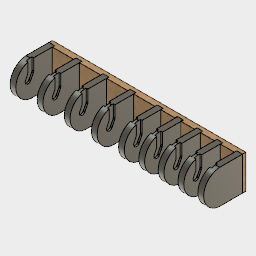
NEW AND IMPROVED Spool Holder x8 v3 (Autodesk Fusion 360 design; units mm, degrees)
Autodesk Fusion 360 part; units mm, degrees
note: some values were not read from the file. Chosen so that the rebuilt part matches the saved one: which face or edge a step refers to. Set by a fixed rule: which sketch regions a step uses.
sketch "Sketch1" plane through (0, 0, 0) normal (0, 1, 0) x (1, 0, 0)
  line L0 (-70, -30) -> (318, -30)
  line L1 (318, -30) -> (318, 40)
  line L2 (318, 40) -> (-70, 40)
  line L3 (-70, 40) -> (-70, -30)
  dimension "d1" = 70
  dimension "d2" = 388
  measures "d1" distance of L0.start L2.end
  measures "d2" distance of L0.start L0.end
extrude "Extrude1" add sketch "Sketch1" along normal blind 9 makes body 1
sketch "Sketch2" plane through (0, 0, 0) normal (0, -1, 0) x (1, 0, 0)
  line L0 (-70, 30) -> (-70, -40)
  line L1 (-70, 30) -> (-64, 30)
  line L2 (-64, 30) -> (-64, -40)
  line L3 (-64, -40) -> (-70, -40)
  line L4 (-70, -40) -> (-70, 30)
  line L5 (-20, 30) -> (-8, 30)
  line L6 (-8, 30) -> (-8, -40)
  line L7 (-8, -40) -> (-20, -40)
  line L8 (-20, -40) -> (-20, 30)
  line L9 (-70, 30) -> (318, 30)
  line L10 (318, -40) -> (-70, -40)
  line L11 (36, 30) -> (48, 30)
  line L12 (48, 30) -> (48, -40)
  line L13 (48, -40) -> (36, -40)
  line L14 (36, -40) -> (36, 30)
  line L15 (92, 30) -> (104, 30)
  line L16 (104, 30) -> (104, -40)
  line L17 (104, -40) -> (92, -40)
  line L18 (92, -40) -> (92, 30)
  line L19 (148, 30) -> (160, 30)
  line L20 (160, 30) -> (160, -40)
  line L21 (160, -40) -> (148, -40)
  line L22 (148, -40) -> (148, 30)
  line L23 (189, 30) -> (201, 30)
  line L24 (201, 30) -> (201, -40)
  line L25 (201, -40) -> (189, -40)
  line L26 (189, -40) -> (189, 30)
  line L27 (230, 30) -> (242, 30)
  line L28 (242, 30) -> (242, -40)
  line L29 (242, -40) -> (230, -40)
  line L30 (230, -40) -> (230, 30)
  line L31 (271, 30) -> (283, 30)
  line L32 (283, 30) -> (283, -40)
  line L33 (283, -40) -> (271, -40)
  line L34 (271, -40) -> (271, 30)
  line L35 (312, 30) -> (318, 30)
  line L36 (318, 30) -> (318, -40)
  line L37 (318, -40) -> (312, -40)
  line L38 (312, -40) -> (312, 30)
  dimension "d15" = 6
  dimension "d22" = 12
  dimension "d23" = 12
  dimension "d24" = 12
  dimension "d25" = 12
  dimension "d26" = 12
  dimension "d27" = 44
  dimension "d28" = 44
  dimension "d29" = 44
  dimension "d30" = 44
  dimension "d31" = 29
  dimension "d32" = 29
  dimension "d33" = 29
  dimension "d34" = 12
  dimension "d35" = 12
  dimension "d36" = 6
  dimension "d37" = 29
  measures "d15" distance of L0.start L1.end
  measures "d22" distance of L5.start L5.end
  measures "d23" distance of L11.start L11.end
  measures "d24" distance of L15.start L15.end
  measures "d25" distance of L19.start L19.end
  measures "d26" distance of L23.start L23.end
  measures "d27" distance of L2 L8
  measures "d28" distance of L6 L14
  measures "d29" distance of L12 L18
  measures "d30" distance of L16 L22
  measures "d31" distance of L20 L26
  measures "d32" distance of L24 L30
  measures "d33" distance of L28 L34
  measures "d34" distance of L28 L30
  measures "d35" distance of L32 L34
  measures "d36" distance of L36 L38
  measures "d37" distance of L32 L38
extrude "Extrude2" cut sketch "Sketch2" against normal blind 5 contours L0 L1 L2 L3 L4 L9 L10 | L5 L6 L7 L8 L9 L10 | L9 L10 L11 L12 L13 L14 | L9 L10 L15 L16 L17 L18 | L9 L10 L19 L20 L21 L22 | L9 L10 L23 L24 L25 L26 | L9 L10 L27 L28 L29 L30 | L9 L10 L31 L32 L33 L34 | L9 L10 L35 L36 L37 L38 bodies 1
extrude "Extrude3" add 1 faces at (-68, 5, -16.6667) along direction (0, -1, 0) blind 100 separate body on bodies 1 makes body 2
sketch "Sketch3" plane through (0, 5, 0) normal (0, -1, 0) x (1, 0, 0)
  line L0 (-8, 30) -> (-20, 30)
  line L1 (-20, 30) -> (-20, -40)
  line L2 (-20, -40) -> (-8, -40)
  line L3 (-8, -40) -> (-8, 30)
  line L4 (-14, 30) -> (-14, -40)
sketch "Sketch4" plane through (-70, 0, 0) normal (-1, 0, 0) x (0, -1, 0)
  line L0 (-5, 30) -> (-5, -40)
  line L1 (-5, -40) -> (95, -40)
  line L2 (95, -40) -> (95, 30)
  line L3 (95, 30) -> (-5, 30)
  line L4 (0, 30) -> (0, -40)
  line L5 (0, -5) -> (44.9994, -5.2262)
  circle A0 centre (44.9994, -5.2262) radius 40
  circle A1 centre (40, -5.1131) radius 35.1778
  point P0 (0, 30)
  point P1 (0, -40)
  dimension "d46" = 45
  dimension "d47" = 80
  dimension "d48" = 40
  measures "d46" distance of L5.start L5.end
  measures "d47" diameter of A0
  measures "d48" distance of L4 A1.centre
extrude "Extrude5" cut sketch "Sketch4" against normal blind 6 contours L1 L3 A0 A1 | L1 L2 L3 A0 picked at (81.0139, 1.7538) bodies 2
sketch "Sketch6" plane through (-70, 0, 0) normal (-1, 0, 0) x (0, -1, 0)
  arc A0 (44.5145, -40) -> (42.133, 30) centre (40, -5.1131) ccw
  line L0 (42.133, 30) -> (-5, 30)
  line L1 (-5, 30) -> (-5, -40)
  line L2 (-5, -40) -> (44.5145, -40)
  line L3 (-5, -5) -> (40, -5)
  circle A1 centre (40, -5) radius 2.5
  dimension "d53" = 45
  dimension "d54" = 5
  measures "d53" distance of L3.start L3.end
  measures "d54" diameter of A1
sketch "Sketch7" plane through (-64, 0, 0) normal (1, 0, 0) x (0, 1, 0)
  arc A0 (-42.133, 30) -> (-44.5145, -40) centre (-40, -5.1131) ccw
  line L0 (-44.5145, -40) -> (5, -40)
  line L1 (5, -40) -> (5, 30)
  line L2 (5, 30) -> (-42.133, 30)
  line L3 (-50, -5) -> (-40, -5) construction
  line L4 (0, -40) -> (0, 30)
  circle A1 centre (-50, -5) radius 40
  circle A2 centre (-45, 3.6603) radius 40
  line L5 (-39, 3.6603) -> (-44.6262, -7.6687)
  line L6 (-51.4175, 5.6353) -> (-55.3738, -2.3313)
  line L7 (-38.3738, 6.329) -> (-38.3738, 51)
  line L8 (-50.3738, 10.0832) -> (-50.3738, 51)
  arc A3 (-39, 3.6603) -> (-38.3738, 6.329) centre (-44.3738, 6.329) ccw
  arc A4 (-55.3738, -2.3313) -> (-44.6262, -7.6687) centre (-50, -5) ccw
  arc A5 (-51.4175, 5.6353) -> (-50.3738, 10.0832) centre (-60.3738, 10.0832) ccw
  dimension "d57" = 12
  dimension "d388" = 50
  dimension "d389" = 80
  dimension "d390" = 80
  dimension "d393" = 10
  measures "d57" diameter of A4
  measures "d388" distance of L3.start L4
  measures "d389" diameter of A1
  measures "d390" diameter of A2
  measures "d393" radius of A5
copy_body "Body->Comp1" bodies 1 removing the originals makes body 3 in component "Backing Board"
sketch "Sketch9" plane through (0, 0, 0) normal (0, -1, 0) x (1, 0, 0)
  line L0 (-20, -40) -> (-20, 30)
  line L1 (-20, 30) -> (-64, 30)
  line L2 (-64, 30) -> (-64, -40)
  line L3 (-64, -40) -> (-20, -40)
  line L4 (-64, -5) -> (-20, -5)
  line L5 (283, 30) -> (283, -40)
  line L6 (312, -40) -> (312, 30)
  line L7 (283, -5) -> (312, -5)
  line L8 (104, 30) -> (104, -40)
  line L9 (148, -40) -> (148, 30)
  line L10 (104, -5) -> (148, -5)
  line L11 (160, 30) -> (160, -40)
  line L12 (189, -40) -> (189, 30)
  line L13 (160, -5) -> (189, -5)
  circle A0 centre (-42, -5) radius 2
  circle A1 centre (126, -5) radius 2
  circle A2 centre (174.5, -5) radius 2
  circle A3 centre (297.5, -5) radius 2
  dimension "d290" = 4
  dimension "d291" = 4
  dimension "d292" = 4
  dimension "d293" = 4
  measures "d290" diameter of A0
  measures "d291" diameter of A1
  measures "d292" diameter of A2
  measures "d293" diameter of A3
extrude "Extrude1'" cut sketch "Sketch9" against normal blind 9 contours L4 A0 | L4 A0 | L7 A3 | L7 A3 | L10 A1 | L10 A1 bodies 3 in component "Backing Board"
extrude "Extrude2'" add 1 faces at (-70, 6.3333, -16.6667) along direction (-1, 0, 0) blind 6 on bodies 3 bodies 3 in component "Backing Board"
extrude "Extrude3'" add 1 faces at (318, 6.3333, 6.6667) along direction (1, 0, 0) blind 6 on bodies 3 bodies 3 in component "Backing Board"
extrude "Extrude11" add 1 faces at (-70, -27.2158, -16.6667) along direction (-1, 0, 0) blind 6 on bodies 2 bodies 2
extrude "Extrude12" cut sketch "Sketch7" against normal blind 3.5 contours A0 L2 L5 L6 L7 L8 A3 A4 A5 bodies 2
sketch "Sketch10" plane through (-76, 0, 0) normal (-1, 0, 0) x (0, -1, 0)
  arc A0 (44.5145, -40) -> (42.133, 30) centre (40, -5.1131) ccw
  line L0 (42.133, 30) -> (-5, 30)
  line L1 (-5, 30) -> (-5, -40)
  line L2 (-5, -40) -> (44.5145, -40)
  arc A1 (44.6262, -7.6687) -> (55.3738, -2.3313) centre (50, -5) ccw
  line L3 (44.6262, -7.6687) -> (39, 3.6603)
  arc A2 (38.3738, 6.329) -> (39, 3.6603) centre (44.3738, 6.329) ccw
  line L4 (38.3738, 6.329) -> (38.3738, 30)
  line L5 (38.3738, 30) -> (42.133, 30)
  arc A3 (50.3738, 28.5003) -> (42.133, 30) centre (40, -5.1131) ccw
  line L6 (50.3738, 28.5003) -> (50.3738, 10.0832)
  arc A4 (50.3738, 10.0832) -> (51.4175, 5.6353) centre (60.3738, 10.0832) ccw
  line L7 (51.4175, 5.6353) -> (55.3738, -2.3313)
extrude "Extrude13" cut sketch "Sketch10" against normal blind 3.5 contours A0 L0 A1 L3 A2 L4 L5 A3 L6 A4 L7 bodies 2
copy_body "CopyPasteBodies1" bodies 2 makes body 4
move_body "Move1" bodies 4 to x (1, 0, 0) y (0, 1, 0) z (0, 0, 1) at (40, 0, 0)
copy_body "CopyPasteBodies3" bodies 2 makes body 5
move_body "Move2" bodies 5 to x (1, 0, 0) y (0, 1, 0) z (0, 0, 1) at (100, 0, 0)
copy_body "Body->Comp4" bodies 2 removing the originals makes body 6 in component "LEFT END"
copy_body "Body->Comp5" bodies 4 removing the originals makes body 7 in component "Center"
copy_body "Body->Comp6" bodies 5 removing the originals makes body 8 in component "RIGHT END"
extrude "Extrude1''" add 1 faces at (-72.5, -43.6269, 15.4707) along direction (-1, 0, 0) blind 3.5 on bodies 6 bodies 6 in component "LEFT END"
extrude "Extrude1'''" add 1 faces at (32.5, -43.6269, 15.4707) along direction (1, 0, 0) blind 3.5 on bodies 8 bodies 8 in component "RIGHT END"
extrude "Extrude4" add 1 faces at (124.6667, 9, 19) along direction (0, 1, 0) blind 3 on bodies 3 bodies 3 in component "Backing Board"
component "Backing Board" placed x (1, 0, 0) y (0, 1, 0) z (0, 0, 1) at (0, 0, 0)
component "LEFT END" placed x (1, 0, 0) y (0, 1, 0) z (0, 0, 1) at (0, 0, 0)
component "Center" placed x (1, 0, 0) y (0, 1, 0) z (0, 0, 1) at (16, 0, 0)
component "RIGHT END" placed x (1, 0, 0) y (0, 1, 0) z (0, 0, 1) at (288, 0, 0)
component "Center" placed x (1, 0, 0) y (0, 1, 0) z (0, 0, 1) at (72, 0, 0)
component "Center" placed x (1, 0, 0) y (0, 1, 0) z (0, 0, 1) at (128, 0, 0)
component "Center" placed x (1, 0, 0) y (0, 1, 0) z (0, 0, 1) at (184, 0, 0)
component "Center" placed x (1, 0, 0) y (0, 1, 0) z (0, 0, 1) at (226, 0, 0)
component "Center" placed x (1, 0, 0) y (0, 1, 0) z (0, 0, 1) at (266, 0, 0)
component "Center" placed x (1, 0, 0) y (0, 1, 0) z (0, 0, 1) at (307, 0, 0)
equation "d2 = overalllength"
equation "ThickPly = 9 mm"
equation "ThinPly = 6 mm"
equation "Space1 = 44 mm"
equation "Space2 = 44 mm"
equation "space3 = 44 mm"
equation "space4 = 44 mm"
equation "space5 = 29 mm"
equation "space6 = 29 mm"
equation "space7 = 29 mm"
equation "space8 = 29 mm"
equation "d15 = ThinPly"
equation "d22 = ThinPly * 2"
equation "d23 = ThinPly * 2"
equation "d24 = ThinPly * 2"
equation "d25 = ThinPly * 2"
equation "d26 = ThinPly * 2"
equation "d27 = Space1"
equation "d28 = Space2"
equation "d29 = space3"
equation "d30 = space4"
equation "d31 = space5"
equation "d32 = space6"
equation "d33 = space7"
equation "d34 = ThinPly * 2"
equation "d35 = ThinPly * 2"
equation "d36 = ThinPly"
equation "d37 = space8"
equation "overalllength = ( Space1 + Space2 + space3 + space4 + space5 + space6 + space7 + space8 ) + ( ThinPly * 2 ) + ( ThinPly * 14 )"
equation "depthsiderail = 80 mm"
equation "d49 = -ThinPly"
equation "d294 = -ThickPly"
